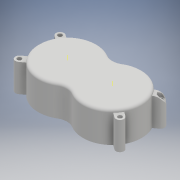
# Autodesk Inventor part: Gehaeuse_V3
Saved by Autodesk Inventor 2017 (Build 210142000, 142)
## iProperties
Created: 2019-05-23
Part Number: Gehaeuse_V3
Material: Generic
Document SubType Name: Modeling
Designer: Ole Simmering
Density: 1 g/cm^3
Appearance: Default
Author: Ole Simmering
Autodesk Inventor part; units mm, degrees
ref_plane "YZ Plane" through (0, 0, 0) normal (1, 0, 0) x (0, 1, 0)
sketch "Sketch1" plane through (0, 0, 0) normal (0, 0, 1) x (1, 0, 0)
  line L0 (-11.999, -0.0009) -> (209.001, -0.0009) construction
  circle A0 centre (47.001, -0.0009) radius 42.5 construction
  circle A1 centre (132.001, -0.0009) radius 42.5 construction
  circle A2 centre (47.001, -0.0009) radius 47.5625 construction
  circle A3 centre (132.001, -0.0009) radius 47.5625 construction
  arc A4 (82.1177, 32.0773) -> (-0.5615, -0.0019) centre (47.001, -0.0009) ccw
  arc A5 (179.5635, -0.0009) -> (96.8843, 32.0773) centre (132.001, -0.0009) ccw
  arc A6 (-0.5615, -0.0019) -> (82.1177, -32.079) centre (47.001, -0.0009) ccw
  arc A7 (96.8843, -32.079) -> (179.5635, -0.0009) centre (132.001, -0.0009) ccw
  arc A8 (75.7238, 47.5616) -> (-8.5615, -0.0015) centre (47.001, -0.0009) ccw
  arc A9 (187.5635, -0.0009) -> (103.2782, 47.5616) centre (132.001, -0.0009) ccw
  line L1 (47.001, 47.5616) -> (132.001, 47.5616) construction
  arc A10 (75.7238, 47.5616) -> (103.2782, 47.5616) centre (89.501, 70.3754) ccw
  arc A11 (-8.5615, -0.0015) -> (75.7238, -47.5634) centre (47.001, -0.0009) ccw
  arc A12 (103.2782, -47.5634) -> (187.5635, -0.0009) centre (132.001, -0.0009) ccw
  arc A13 (103.2782, -47.5634) -> (75.7238, -47.5634) centre (89.501, -70.3772) ccw
  arc A14 (82.1177, 32.0773) -> (96.8843, 32.0773) centre (89.501, 38.8217) ccw
  line L2 (82.1177, 32.0773) -> (96.8843, 32.0773) construction
  arc A15 (96.8843, -32.079) -> (82.1177, -32.079) centre (89.501, -38.8234) ccw
  point P0 (89.501, 21.3519)
  point P1 (46.9513, 55.5616)
  point P2 (132.0501, 55.5616)
  dimension "d5" = 221
  dimension "d6" = 85
  dimension "d7" = 85
  dimension "d8" = 85
  dimension "d9" = 95.125
  dimension "d10" = 95.125
  dimension "d12" = 8
  dimension "d20" = 10
  constraints: 36 point on circle, 16 centre point, 6 end point, 6 symmetric about line, 5 point on line, 5 tangent, 3 horizontal, 2 coincident, 2 concentric, 7 other
  measures "d5" distance of L0.start L0.end
  measures "d6" diameter of A0
  measures "d7" diameter of A1
  measures "d8" distance of A1.centre A0.centre
  measures "d9" diameter of A2
  measures "d10" diameter of A3
  measures "d12" radial gap between concentric circles of A4 A8
  measures "d20" radius of A14
extrude "Extrusion1" add sketch "Sketch1" along normal blind 50
sketch "Sketch2" plane through (0, 0, 50) normal (0, 0, 1) x (1, 0, 0)
  arc A0 (75.7238, 47.5616) -> (75.7238, -47.5634) centre (47.001, -0.0009) ccw projected
  arc A1 (75.7238, 47.5616) -> (103.2782, 47.5616) centre (89.501, 70.3754) ccw projected
  arc A2 (103.2782, -47.5634) -> (103.2782, 47.5616) centre (132.001, -0.0009) ccw projected
  arc A3 (103.2782, -47.5634) -> (75.7238, -47.5634) centre (89.501, -70.3772) ccw projected
  point P0 (0, 0)
extrude "Extrusion2" add sketch "Sketch2" along normal blind 8
fillet "Fillet1" radius 5 4 edges at (89.501, -43.7261, 58) (187.5635, -0.0009, 58) (89.501, 43.7243, 58) (-8.5615, -0.0009, 58)
sketch "Sketch8" plane through (0, 0, 0) normal (0, 0, -1) x (-1, 0, 0)
  arc A0 (-75.7238, -47.5634) -> (-75.7238, 47.5616) centre (-47.001, -0.0009) ccw construction
  arc A1 (-103.2782, 47.5616) -> (-75.7238, 47.5616) centre (-89.501, 70.3754) ccw construction
  arc A2 (-103.2782, 47.5616) -> (-103.2782, -47.5634) centre (-132.001, -0.0009) ccw construction
  arc A3 (-75.7238, -47.5634) -> (-103.2782, -47.5634) centre (-89.501, -70.3772) ccw construction
  circle A4 centre (-89.501, -0.0009) radius 110.5 construction
  line L0 (-180.9153, 26.354) -> (-189.409, 32.5416)
  arc A5 (-180.5767, 44.6656) -> (-189.409, 32.5416) centre (-184.9929, 38.6036) ccw
  line L1 (-180.5767, 44.6656) -> (-172.083, 38.4779)
  line L2 (-184.9929, 38.6036) -> (-176.9102, 32.7154) construction
  line L3 (-273, -0.0009) -> (56, -0.0009) construction
  line L4 (-89.501, 70.3754) -> (-89.501, -70.3772) construction
  circle A6 centre (-184.9929, 38.6036) radius 4
  arc A7 (-172.083, 38.4779) -> (-180.9153, 26.354) centre (-132.001, -0.0009) ccw
  line L5 (1.9134, 26.354) -> (10.407, 32.5416)
  arc A8 (10.407, 32.5416) -> (1.5747, 44.6656) centre (5.9909, 38.6036) ccw
  line L6 (1.5747, 44.6656) -> (-6.9189, 38.4779)
  line L7 (5.9909, 38.6036) -> (-2.0918, 32.7154) construction
  circle A9 centre (5.9909, 38.6036) radius 4
  arc A10 (1.9134, 26.354) -> (-6.9189, 38.4779) centre (-47.001, -0.0009) ccw
  line L8 (-180.9153, -26.3557) -> (-189.409, -32.5433)
  arc A11 (-189.409, -32.5433) -> (-180.5767, -44.6673) centre (-184.9929, -38.6053) ccw
  line L9 (-180.5767, -44.6673) -> (-172.083, -38.4797)
  line L10 (-184.9929, -38.6053) -> (-176.9102, -32.7171) construction
  circle A12 centre (-184.9929, -38.6053) radius 4
  arc A13 (-180.9153, -26.3557) -> (-172.083, -38.4797) centre (-132.001, -0.0009) ccw
  line L11 (1.5747, -44.6673) -> (-6.9189, -38.4797)
  line L12 (5.9909, -38.6053) -> (-2.0918, -32.7171) construction
  arc A14 (-6.9189, -38.4797) -> (1.9134, -26.3557) centre (-47.001, -0.0009) ccw
  circle A15 centre (5.9909, -38.6053) radius 4
  line L13 (1.9134, -26.3557) -> (10.407, -32.5433)
  arc A16 (1.5747, -44.6673) -> (10.407, -32.5433) centre (5.9909, -38.6053) ccw
  point P0 (0, 0)
  point P1 (-89.501, -0.0009)
  dimension "d39" = 221
  dimension "d40" = 15
  dimension "d42" = 10
  dimension "d43" = 8
  constraints: 28 end point, 22 symmetric about line, 19 point on circle, 13 centre point, 6 coincident, 3 tangent, 2 parallel, 1 horizontal, 1 line through centre, 1 midpoint, 1 point on line, 1 vertical, 9 other
  measures "d39" diameter of A4
  measures "d40" distance between parallel lines of L1 L0
  measures "d42" distance of L2.end L2.start
  measures "d43" diameter of A6
extrude "Extrusion4" add sketch "Sketch8" against normal blind 53
ref_plane "Work Plane1" through (176.4992, 32.416, 53) normal (-0.5888191, 0.8082649, 0) x (0.8082649, 0.5888191, 0)
sketch "Sketch9" plane through (176.4992, 32.416, 53) normal (-0.5888191, 0.8082649, 0) x (0.8082649, 0.5888191, 0)
  line L0 (18.0085, 53) -> (18.0085, 0) construction
  line L1 (18.0085, 0) -> (18.0085, 53) construction
  line L2 (18.0078, 17.6544) -> (26.4514, 17.6544)
  line L3 (26.4514, 17.6544) -> (26.4514, -7)
  line L4 (26.4514, -7) -> (0.5085, -7)
  line L5 (0.5085, -7) -> (0.5085, 0)
  line L6 (0, 0) -> (0.5085, 0) construction
  line L7 (0.5085, 0) -> (19.7694, 0) construction
  arc A0 (0.5085, 0) -> (18.0078, 17.6544) centre (0.5085, 17.5) ccw
  line L8 (-55.054, 65) -> (-55.054, -19) projected
  point P0 (-161.7452, 53)
  dimension "d46" = 8.4436
  dimension "d47" = 24.6544
  dimension "d48" = 25.9429
  dimension "d49" = 7
  constraints: 12 end point, 2 horizontal, 2 perpendicular, 2 point on circle, 2 point on line, 2 tangent, 1 centre point
  measures "d46" distance of L2.start L2.end
  measures "d47" distance of L2.end L3.end
  measures "d48" distance of L3.end L4.end
  measures "d49" distance of L4.end L5.end
revolve "Revolution1" cut sketch "Sketch9" angle 20 mid plane about axis through (132.001, -0.0009, 0) along (0, 0, 1)
ref_plane "Work Plane2" through (0, 0, 53) normal (0, 0, -1) x (-1, 0, 0)
sketch "Sketch11" plane through (0, 0, 53) normal (0, 0, -1) x (-1, 0, 0)
  line L0 (-189.409, 32.5416) -> (-180.9153, 26.354) construction
  line L1 (-172.083, 38.4779) -> (-180.5767, 44.6656) construction
  arc A0 (-172.083, 38.4779) -> (-180.9153, 26.354) centre (-132.001, -0.0009) ccw construction
  circle A1 centre (-184.9929, 38.6036) radius 4 projected
  line L2 (-182.2729, 33.5109) -> (-188.0432, 33.7017)
  line L3 (-188.0432, 33.7017) -> (-190.7632, 38.7943)
  line L4 (-190.7632, 38.7943) -> (-187.7128, 43.6962)
  line L5 (-187.7128, 43.6962) -> (-181.9425, 43.5055)
  line L6 (-181.9425, 43.5055) -> (-179.2225, 38.4128)
  line L7 (-179.2225, 38.4128) -> (-182.2729, 33.5109)
  point P0 (0, 0)
  dimension "d52" = 10
  constraints: 12 end point, 1 coincident, 17 other
  measures "d52" distance between parallel lines of L4 L7
extrude "Extrusion5" cut sketch "Sketch11" along normal blind 10
equation "\"d7\" = d6"
equation "\"d8\" = d6"
equation "\"d10\" = d9"
body "Solid1"
